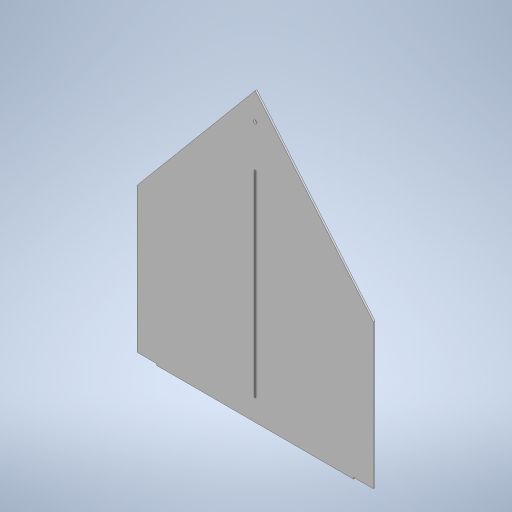
# Autodesk Inventor part: side
Saved by Autodesk Inventor 2023 (Build 270158000, 158)
## iProperties
Created: 2023-10-15
Part Number: side
Material: Generic
Document SubType Name: Modeling
Designer: Nate
Density: 1 g/cm^3
Appearance: Default
Author: Nate
Autodesk Inventor part; units mm, degrees
ref_plane "YZ Plane" through (0, 0, 0) normal (1, 0, 0) x (0, 1, 0)
ref_plane "XZ Plane" through (0, 0, 0) normal (0, 1, 0) x (-1, 0, 0)
ref_plane "XY Plane" through (0, 0, 0) normal (0, 0, 1) x (1, 0, 0)
sketch "Sketch1" plane through (0, 0, 0) normal (0, 0, 1) x (1, 0, 0)
  line L0 (0, 0) -> (-3.175, 0)
  line L1 (-3.175, 0) -> (-3.175, 381)
  line L2 (-3.175, 381) -> (0, 381)
  line L3 (0, 381) -> (0, 0)
  line L4 (-3.175, -38.1) -> (-555.625, -38.1)
  line L5 (-555.625, -38.1) -> (-555.625, 419.1)
  line L6 (-555.625, 419.1) -> (-3.175, 419.1)
  line L7 (-3.175, 419.1) -> (-3.175, -38.1)
  line L8 (-555.625, 190.5) -> (-282.575, -38.1)
  line L9 (-555.625, 190.5) -> (-282.575, 419.1)
  circle A0 centre (-503.174, 190.5) radius 3.175
  line L10 (-41.275, 188.9125) -> (-422.275, 188.9125)
  line L11 (-422.275, 188.9125) -> (-422.275, 192.0875)
  line L12 (-422.275, 192.0875) -> (-41.275, 192.0875)
  line L13 (-41.275, 192.0875) -> (-41.275, 188.9125)
  point P0 (-1.5875, 0)
  point P1 (-3.175, 0)
  point P2 (-3.175, 381)
  point P3 (-41.275, 190.5)
  dimension "d0" = 3.175
  dimension "d1" = 381
  dimension "d2" = 552.45
  dimension "d3" = 457.2
  dimension "d4" = 38.1
  dimension "d5" = 228.6
  dimension "d6" = 279.4
  dimension "d7" = 228.6
  dimension "d9" = 6.35
  dimension "d10" = 228.6
  dimension "d11" = 499.999
  dimension "d12" = 279.4
  dimension "d15" = 381
  dimension "d16" = 3.175
  dimension "d17" = 227.0125
  dimension "d18" = 38.1
  constraints: 28 end point, 6 parallel, 3 horizontal, 3 midpoint, 3 perpendicular, 3 point on line, 1 centre point
  measures "d0" distance of L1.end L2.end
  measures "d1" distance of L0.end L1.end
  measures "d2" distance of L5.end L6.end
  measures "d3" distance between parallel lines of L6 L4
  measures "d4" distance from line of L4 point (-1.588, 0)
  measures "d5" distance from line of L8.start L4
  measures "d6" distance from line of L1 L8.end
  measures "d7" distance from line of L6 L8.start
  measures "d9" diameter of A0
  measures "d10" distance from line of L6 A0.centre
  measures "d11" distance from line of L1 A0.centre
  measures "d12" distance from line of L7 L9.end
  measures "d15" distance of L11.end L12.end
  measures "d16" distance between parallel lines of L12 L10
  measures "d17" distance between parallel lines of L10 L4
  measures "d18" distance from line of point (-41.275, 190.5) L7
extrude "Extrusion1" add sketch "Sketch1" along normal blind 3.175 contours L0 L1 L2 L3 | L7 L4 L8 L9 L6 L1
move or copy body "Move Body1" bodies to move or copy 1 copy no rotation origin (0, 0, 0) rotation axis (0, 0, 1) rotation angle -90
move or copy body "Move Body2" bodies to move or copy 1 copy no translate (25.4, 0, 0)
body "Solid1"
